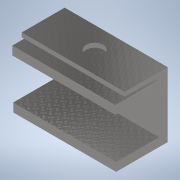
# Autodesk Inventor part: Clamp for Box Crusher
Saved by Autodesk Inventor 2021 (Build 250183000, 183)
## iProperties
Created: 2021-03-08
Part Number: Clamp for Box Crusher
Material: Generic
Document SubType Name: Modeling
Designer: david
Density: 1 g/cm^3
Appearance: Diamond Plate
Author: david
Autodesk Inventor part; units mm, degrees
ref_plane "YZ Plane" through (0, 0, 0) normal (1, 0, 0) x (0, 1, 0)
ref_plane "XZ Plane" through (0, 0, 0) normal (0, 1, 0) x (-1, 0, 0)
ref_plane "XY Plane" through (0, 0, 0) normal (0, 0, 1) x (1, 0, 0)
sketch "Sketch1" plane through (0, 0, 0) normal (1, 0, 0) x (0, 1, 0)
  line L0 (27.6225, -46.0375) -> (27.6225, -109.5375)
  line L1 (27.6225, -109.5375) -> (88.5825, -109.5375)
  line L2 (14.9225, -46.0375) -> (14.9225, -122.2375)
  line L3 (14.9225, -122.2375) -> (104.7551, -122.2375)
  line L4 (27.6225, -46.0375) -> (14.9225, -46.0375)
  line L5 (88.5825, -109.5375) -> (104.7551, -109.5375)
  line L6 (101.2825, -44.7675) -> (88.5825, -44.7675)
  line L7 (88.5825, -44.7675) -> (88.5825, -108.2675)
  line L8 (88.5825, -108.2675) -> (101.2825, -108.2675)
  line L9 (101.2825, -108.2675) -> (101.2825, -44.7675)
  line L10 (111.1051, -58.7375) -> (104.7551, -58.7375)
  line L11 (104.7551, -58.7375) -> (104.7551, -109.5375)
  line L12 (104.7551, -122.2375) -> (111.1051, -122.2375)
  line L13 (111.1051, -122.2375) -> (111.1051, -58.7375)
  point P0 (0, 0)
  dimension "d2" = 12.7
  dimension "d4" = 63.5
  dimension "d7" = 63.5
  dimension "d8" = 12.7
  dimension "d9" = 1.27
  dimension "d10" = 60.96
  dimension "d11" = 6.35
  dimension "d12" = 63.5
  constraints: 28 end point, 4 parallel, 3 horizontal, 3 perpendicular
  measures "d2" distance between parallel lines of L1 L3
  measures "d4" distance of L0.start L0.end
  measures "d7" distance of L8.end L6.start
  measures "d8" distance of L6.start L6.end
  measures "d9" distance between parallel lines of L8 L5
  measures "d10" distance of L0.end L1.end
  measures "d11" distance of L10.start L10.end
  measures "d12" distance of L12.end L10.start
extrude "Extrusion1" add sketch "Sketch1" along normal blind 152.4
sketch "Sketch2" plane through (0, 111.1051, -58.7375) normal (0, 1, 0) x (1, 0, 0)
  circle A0 centre (76.2, 31.75) radius 12.7
  line L0 (0, 63.5) -> (152.4, 63.5) projected
  line L1 (0, 63.5) -> (0, 0) projected
  line L2 (152.4, 63.5) -> (152.4, 0) projected
  point P0 (0, -58.7375)
  dimension "d16" = 152.4
  dimension "d17" = 76.2
  dimension "d18" = 63.5
  dimension "d19" = 31.75
  dimension "d20" = 25.4
  constraints: 1 centre point
  measures "d16" distance of L0.start L0.end
  measures "d17" distance from line of A0.centre L1
  measures "d18" distance of L0.end L2.end
  measures "d19" distance from line of A0.centre L0
  measures "d20" diameter of A0
extrude "Extrusion2" cut sketch "Sketch2" against normal blind 7.62
equation "\"d17\" = 0.5 * d16"
equation "\"d19\" = 0.5 * d18"
body "Solid1"
